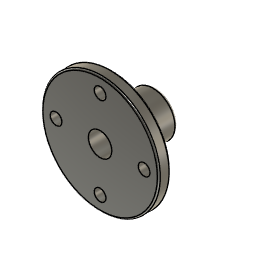
Motor Hub_ (Autodesk Fusion 360 design; units mm, degrees)
Autodesk Fusion 360 part; units mm, degrees
sketch "Sketch1" plane through (0, 0, 0) normal (0, 1, 0) x (1, 0, 0)
  circle A0 centre (0, 0) radius 4
  circle A1 centre (0, 0) radius 7.5
  circle A2 centre (0, 0) radius 20
  circle A3 centre (0, 0) radius 15 construction
  circle A4 centre (0, -15) radius 2
  circle A5 centre (15, 0) radius 2
  circle A6 centre (0, 15) radius 2
  circle A7 centre (-15, 0) radius 2
  dimension "d1" = 8
  dimension "d2" = 15
  dimension "d3" = 40
  dimension "d4" = 4
  dimension "d6" = 360
  constraint coincident A0.centre A1.centre
  constraint concentric A0 A1
  constraint concentric A1 A2
  constraint concentric A2 A3
  constraint coincident A3 A4.centre
  measures "d1" diameter of A0
  measures "d2" diameter of A1
  measures "d3" diameter of A2
  measures "d4" diameter of A4
extrude "Extrude1" add sketch "Sketch1" along normal blind 15 contours A1
extrude "Extrude2" add sketch "Sketch1" against normal blind 4 contours A1 | A2
fillet "Fillet1" radius 0.5 2 edges at (-18.6465, -4, -7.2323) (-18.6465, 0, 7.2323)
fillet "Fillet2" radius 1 2 edges at (-6.9925, 0, 2.7121) (-6.9925, 15, 2.7121)
hole "Hole1" at (0, 7.8114, 7.5) direction (0, 0, -1) diameter 3.332 depth 8 tip angle 118
thread "Thread1" "ISO Metric profile 4.0 M4x0.7 M4x0.7 6H" thread offset 0 thread depth 7.4
